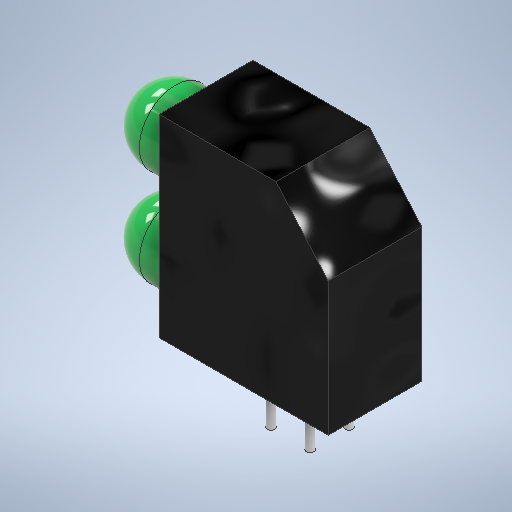
# Autodesk Inventor part: SSF-LXHM250GGD
Saved by Autodesk Inventor 2025 (Build 290162000, 162)
## iProperties
Created: 2026-07-27
Part Number: SSF-LXHM250GGD
Material: Generic
Document SubType Name: Modeling
Designer: tapen
Density: 1 g/cm^3
Appearance: Default
Author: tapen
Autodesk Inventor part; units mm, degrees
ref_plane "YZ Plane" through (0, 0, 0) normal (1, 0, 0) x (0, 1, 0)
ref_plane "XZ Plane" through (0, 0, 0) normal (0, 1, 0) x (-1, 0, 0)
ref_plane "XY Plane" through (0, 0, 0) normal (0, 0, 1) x (1, 0, 0)
sketch "Sketch1" plane through (0, 0, 0) normal (0, 0, 1) x (1, 0, 0)
  line L0 (0, 0) -> (11, 0)
  line L1 (11, 0) -> (11, 8.7)
  line L2 (0, 0) -> (0, 12.6)
  line L3 (0, 12.6) -> (7.6, 12.6)
  line L4 (7.6, 12.6) -> (11, 8.7)
  dimension "d0" = 11
  dimension "d1" = 8.7
  dimension "d2" = 12.6
  dimension "d3" = 7.6
  constraints: 10 end point, 2 horizontal, 2 vertical
  measures "d0" distance of L0.start L0.end
  measures "d1" distance of L0.end L1.end
  measures "d2" distance of L0.start L2.end
  measures "d3" distance of L2.end L3.end
extrude "Extrusion1" add sketch "Sketch1" along normal blind 6.1
ref_plane "Work Plane1" through (0, 0, 3.05) normal (0, 0, 1) x (1, 0, 0)
sketch "Sketch2" plane through (0, 0, 3.05) normal (0, 0, 1) x (1, 0, 0)
  line L0 (0, 12.6) -> (0, 0) projected
  line L1 (0, 9.37) -> (-4.5, 9.37)
  line L2 (7.6, 12.6) -> (0, 12.6) projected
  line L3 (0, 11.72) -> (-2, 11.72)
  arc A0 (-2, 11.72) -> (-4.5, 9.37) centre (-2, 9.2152) ccw
  line L4 (0, 9.37) -> (0, 11.72)
  line L5 (0, 12.6) -> (0, 0) projected
  dimension "d6" = 3.23
  dimension "d7" = 4.5
  dimension "d8" = 2.35
  dimension "d10" = 2
  constraints: 6 end point, 2 point on circle, 2 point on line, 1 centre point, 1 horizontal, 1 perpendicular, 1 tangent, 1 vertical
  measures "d6" distance between parallel lines of L2 L1
  measures "d7" distance of L1.start L1.end
  measures "d8" distance between parallel lines of L3 L1
  measures "d10" distance of L3.start L3.end
revolve "Revolution1" add sketch "Sketch2" angle 360 about axis through (0, 9.37, 3.05) along (-1, 0, 0)
ref_plane "Work Plane2" through (0, 6.195, 0) normal (0, 1, 0) x (1, 0, 0)
mirror "Mirror1" about plane through (0, 6.195, 0) normal (0, 1, 0) of "Revolution1"
sketch "Sketch3" plane through (0, 0, 0) normal (0, -1, 0) x (1, 0, 0)
  circle A0 centre (5.5, 1.78) radius 0.25
  line L0 (0, 0) -> (0, 6.1) projected
  line L1 (0, 0) -> (11, 0) construction
  line L2 (0, 0) -> (11, 0)
  circle A1 centre (8.04, 1.78) radius 0.25
  line L3 (2.54, 0) -> (13.54, 0)
  circle A2 centre (5.5, 4.32) radius 0.25
  line L4 (0, 2.54) -> (11, 2.54)
  circle A3 centre (8.04, 4.32) radius 0.25
  line L5 (2.54, 2.54) -> (13.54, 2.54)
  point P0 (0, 3.05)
  point P1 (0, 3.05)
  dimension "d13" = 5.5
  dimension "d15" = 1.27
  dimension "d16" = 0.5
  dimension "d19" = 2.54
  dimension "d22" = 2.54
  constraints: 8 end point, 4 centre point, 2 horizontal, 2 midpoint, 1 vertical, 15 other
  measures "d13" distance from line of A0.centre L0
  measures "d15" vertical distance of point (0, 3.05) A0.centre
  measures "d16" diameter of A0
  measures "d19" distance of A0.centre A1.centre
  measures "d22" distance of A0.centre A2.centre
extrude "Extrusion2" add sketch "Sketch3" along normal blind 3.18
body "Solid1"
